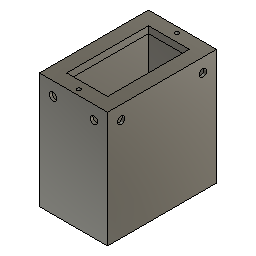
PEM_housing v3 (Autodesk Fusion 360 design; units mm, degrees)
Autodesk Fusion 360 part; units mm, degrees
sketch "Sketch1" plane through (0, 0, 0) normal (0, 0, 1) x (1, 0, 0)
  line L0 (0, 0) -> (50, 0)
  line L1 (50, 0) -> (50, 80)
  line L2 (50, 80) -> (0, 80)
  line L3 (0, 80) -> (0, 0)
  dimension "d1" = 50
  dimension "d2" = 80
  constraint horizontal L0
  constraint vertical L1
  constraint horizontal L2
  constraint vertical L3
  constraint coincident L0.start L3.end
  measures "d1" distance of L0.start L0.end
  measures "d2" distance of L0.start L2.end
extrude "Extrude1" add sketch "Sketch1" along normal blind 5
sketch "Sketch2" plane through (0, 0, 5) normal (0, 0, 1) x (-1, 0, 0)
  line L0 (0, -80) -> (0, 0)
  line L1 (0, 0) -> (-50, 0)
  line L2 (-50, 0) -> (-50, -80)
  line L3 (-50, -80) -> (0, -80)
  line L4 (-40, -10) -> (-10, -10)
  line L5 (-10, -10) -> (-10, -70)
  line L6 (-10, -70) -> (-40, -70)
  line L7 (-40, -70) -> (-40, -10)
  line L8 (-40, -10) -> (-10, -70) construction
  line L9 (-10, -10) -> (-40, -70) construction
  point P0 (-25, -40)
  point P1 (-25, -40)
  dimension "d5" = 30
  dimension "d6" = 60
  constraint horizontal L4
  constraint perpendicular L4 L5
  constraint parallel L4 L6
  constraint parallel L5 L7
  constraint coincident L8 P1
  constraint coincident L9 P1
  constraint coincident P1 P0
  measures "d5" distance of L5.end L6.end
  measures "d6" distance of L4.end L5.end
extrude "Extrude2" cut sketch "Sketch2" against normal blind 6 contours L4 L5 L6 L7
sketch "Sketch3" plane through (0, 0, 5) normal (0, 0, 1) x (-1, 0, 0)
  line L0 (-10, -10) -> (-10, -70)
  line L1 (-10, -70) -> (-40, -70)
  line L2 (-40, -70) -> (-40, -10)
  line L3 (-40, -10) -> (-10, -10)
  line L4 (0, -80) -> (0, 0)
  line L5 (0, 0) -> (-50, 0)
  line L6 (-50, 0) -> (-50, -80)
  line L7 (-50, -80) -> (0, -80)
  point P0 (-25, -76)
  point P1 (-25, -4)
  constraint vertical P0 P1
hole "Hole1" at (25, 76, 5) at (25, 4, 5) direction (0, 0, -1) diameter 2.75 depth 15 tip angle 118
sketch "Sketch4" plane through (0, 0, 0) normal (0, 0, -1) x (1, 0, 0)
  circle A0 centre (25, -76) radius 1.375
  circle A1 centre (25, -4) radius 1.375
  line L0 (10, -70) -> (10, -10)
  line L1 (10, -10) -> (40, -10)
  line L2 (40, -10) -> (40, -70)
  line L3 (40, -70) -> (10, -70)
  line L4 (0, 0) -> (0, -80)
  line L5 (0, -80) -> (50, -80)
  line L6 (50, -80) -> (50, 0)
  line L7 (50, 0) -> (0, 0)
  line L8 (48, -2) -> (2, -2)
  line L9 (2, -2) -> (2, -78)
  line L10 (2, -78) -> (48, -78)
  line L11 (48, -78) -> (48, -2)
  constraint horizontal L8
  constraint vertical L9
  constraint horizontal L10
  constraint vertical L11
extrude "Extrude3" add sketch "Sketch4" along normal blind 80 contours L4 L5 L6 L7
sketch "Sketch5" plane through (0, 0, 0) normal (-1, 0, 0) x (0, -1, 0)
  line L0 (0, -80) -> (0, 5)
  line L1 (0, 5) -> (-80, 5)
  line L2 (-80, 5) -> (-80, -80)
  line L3 (-80, -80) -> (0, -80)
  point P0 (-10, -5)
  point P1 (-70, -5)
  constraint horizontal P0 P1
hole "Hole2" at (0, 10, -5) at (0, 70, -5) direction (1, 0, 0) diameter 5.5 depth 100 tip angle 118
sketch "Sketch6" plane through (0, 80, 0) normal (0, 1, 0) x (-1, 0, 0)
  line L0 (0, -80) -> (0, 5)
  line L1 (0, 5) -> (-50, 5)
  line L2 (-50, 5) -> (-50, -80)
  line L3 (-50, -80) -> (0, -80)
  point P0 (-10, -5)
  point P1 (-40, -5)
  constraint horizontal P0 P1
hole "Hole3" at (40, 80, -5) at (10, 80, -5) direction (0, -1, 0) diameter 5.5 depth 100 tip angle 118
sketch "Sketch7" plane through (0, 78, 0) normal (0, -1, 0) x (1, 0, 0)
  circle A0 centre (40, -5) radius 2.75
  circle A1 centre (10, -5) radius 2.75
  line L0 (48, 0) -> (2, 0)
  line L1 (2, 0) -> (2, -80)
  line L2 (2, -80) -> (48, -80)
  line L3 (48, -80) -> (48, 0)
  line L4 (30, -80) -> (20, -80)
  line L5 (20, -80) -> (20, -70)
  line L6 (20, -70) -> (30, -70)
  line L7 (30, -70) -> (30, -80)
  dimension "d20" = 10
  dimension "d21" = 10
  constraint horizontal L4
  constraint vertical L5
  constraint horizontal L6
  constraint vertical L7
  constraint coincident L2 L4.start
  measures "d20" distance of L4.start L4.end
  measures "d21" distance of L4.start L6.end
extrude "Extrude4" add sketch "Sketch7" along normal blind 10 contours L2 L4 L5 L6 L7
sketch "Sketch8" plane through (0, 2, 0) normal (0, 1, 0) x (-1, 0, 0)
  circle A0 centre (-40, -5) radius 2.75
  circle A1 centre (-10, -5) radius 2.75
  line L0 (-2, 0) -> (-48, 0)
  line L1 (-48, 0) -> (-48, -80)
  line L2 (-48, -80) -> (-2, -80)
  line L3 (-2, -80) -> (-2, 0)
  line L4 (-20, -80) -> (-30, -80)
  line L5 (-30, -80) -> (-30, -70)
  line L6 (-30, -70) -> (-20, -70)
  line L7 (-20, -70) -> (-20, -80)
  dimension "d24" = 10
  dimension "d25" = 10
  constraint horizontal L4
  constraint vertical L5
  constraint horizontal L6
  constraint vertical L7
  constraint coincident L2 L4.start
  measures "d24" distance of L4.start L4.end
  measures "d25" distance of L4.start L6.end
extrude "Extrude5" add sketch "Sketch8" along normal blind 10 contours L2 L4 L5 L6 L7
sketch "Sketch9" plane through (0, 0, -80) normal (0, 0, -1) x (1, 0, 0)
  line L0 (48, -2) -> (48, -78)
  line L1 (48, -78) -> (30, -78)
  line L2 (30, -78) -> (30, -68)
  line L3 (30, -68) -> (20, -68)
  line L4 (20, -68) -> (20, -78)
  line L5 (20, -78) -> (2, -78)
  line L6 (2, -78) -> (2, -2)
  line L7 (2, -2) -> (20, -2)
  line L8 (20, -2) -> (20, -12)
  line L9 (20, -12) -> (30, -12)
  line L10 (30, -12) -> (30, -2)
  line L11 (30, -2) -> (48, -2)
  line L12 (50, 0) -> (0, 0)
  line L13 (0, 0) -> (0, -80)
  line L14 (0, -80) -> (50, -80)
  line L15 (50, -80) -> (50, 0)
  line L16 (1, -1) -> (49, -1)
  line L17 (49, -1) -> (49, -79)
  line L18 (49, -79) -> (1, -79)
  line L19 (1, -79) -> (1, -1)
  constraint horizontal L16
  constraint vertical L17
  constraint horizontal L18
  constraint vertical L19
extrude "Extrude6" cut sketch "Sketch9" against normal blind 2 contours L16 L17 L18 L19
sketch "Sketch10" plane through (0, 0, -78) normal (0, 0, -1) x (1, 0, 0)
  line L0 (30, -12) -> (30, -2)
  line L1 (30, -2) -> (48, -2)
  line L2 (48, -2) -> (48, -78)
  line L3 (48, -78) -> (30, -78)
  line L4 (30, -78) -> (30, -68)
  line L5 (30, -68) -> (20, -68)
  line L6 (20, -68) -> (20, -78)
  line L7 (20, -78) -> (2, -78)
  line L8 (2, -78) -> (2, -2)
  line L9 (2, -2) -> (20, -2)
  line L10 (20, -2) -> (20, -12)
  line L11 (20, -12) -> (30, -12)
  line L12 (1, -79) -> (49, -79)
  line L13 (49, -79) -> (49, -1)
  line L14 (49, -1) -> (1, -1)
  line L15 (1, -1) -> (1, -79)
  point P0 (25, -7)
  point P1 (25, -73)
  constraint vertical P0 P1
hole "Hole4" at (25, 7, -78) at (25, 73, -78) direction (0, 0, 1) diameter 2.75 depth 11 tip angle 180
